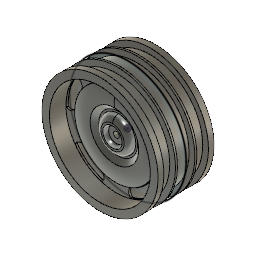
Primeira Modelagem (Autodesk Fusion 360 design; units mm, degrees)
Autodesk Fusion 360 part; units mm, degrees
sketch "Sketch1" plane through (0, 0, 0) normal (0, 1, 0) x (1, 0, 0)
  circle A0 centre (0, 0) radius 3
  dimension "d1" = 6
  constraint coincident A0.centre origin
  measures "d1" diameter of A0
sketch "Sketch1 (2)" plane through (0, 0, 0) normal (1, 0, 0) x (0, 1, 0) in component "roda"
  line L0 (0, -3) -> (0, 3)
  line L1 (-1.4737, 3.362) -> (1.4263, 3.362)
  line L2 (0, 2.7) -> (0.45, 2.7)
  line L3 (0.45, 2.7) -> (0.45, 3)
  line L4 (0.45, 3) -> (0.55, 3)
  line L5 (0.55, 3) -> (0.55, 2.7)
  line L6 (0.55, 2.7) -> (1.15, 2.7)
  line L7 (1.15, 2.7) -> (1.15, 3)
  line L8 (1.15, 3) -> (1.45, 3)
  line L9 (1.45, 3) -> (1.45, 2.6)
  line L10 (1.45, 2.6) -> (0, 2.6)
  line L11 (-0.45, 2.7) -> (-0.45, 3)
  line L12 (-0.45, 3) -> (-0.55, 3)
  line L13 (-0.55, 3) -> (-0.55, 2.7)
  line L14 (-0.55, 2.7) -> (-1.15, 2.7)
  line L15 (-1.15, 2.7) -> (-1.15, 3)
  line L16 (-1.15, 3) -> (-1.45, 3)
  line L17 (-1.45, 3) -> (-1.45, 2.6)
  line L18 (0, 2.7) -> (-0.45, 2.7)
  line L19 (-1.45, 2.6) -> (0, 2.6)
  dimension "d5" = 2.9
  dimension "d6" = 0.45
  dimension "d7" = 0.3
  dimension "d8" = 0.1
  dimension "d9" = 0.3
  dimension "d10" = 0.6
  dimension "d11" = 0.3
  dimension "d12" = 0.3
  dimension "d13" = 0.4
  dimension "d14" = 1.45
  constraint horizontal L1
  constraint coincident L0 L2.start
  constraint perpendicular L0 L2
  constraint perpendicular L2 L3
  constraint perpendicular L3 L4
  constraint perpendicular L4 L5
  constraint perpendicular L5 L6
  constraint perpendicular L6 L7
  constraint perpendicular L7 L8
  constraint perpendicular L8 L9
  constraint perpendicular L0 L10
  constraint symmetric L0 L2.start L18.start
  constraint symmetric L0 L2.end L11.start
  constraint symmetric L0 L3.end L11.end
  constraint symmetric L0 L4.end L12.end
  constraint symmetric L0 L5.end L13.end
  constraint symmetric L0 L6.end L14.end
  constraint symmetric L0 L7.end L15.end
  constraint symmetric L0 L8.end L16.end
  constraint symmetric L0 L9.end L17.end
  constraint symmetric L0 L10.end L19.end
  measures "d5" distance of L1.start L1.end
  measures "d6" distance of L2.start L2.end
  measures "d7" distance of L2.end L3.end
  measures "d8" distance of L3.end L4.end
  measures "d9" distance of L4.end L5.end
  measures "d10" distance of L5.end L6.end
  measures "d11" distance of L6.end L7.end
  measures "d12" distance of L7.end L8.end
  measures "d13" distance of L8.end L9.end
  measures "d14" distance of L9.end L10.end
revolve "Revolve1" add sketch "Sketch1 (2)" angle 360 about axis through (0, 1.75, 0) along (0, 1, 0) contours L0 L11 L12 L13 L14 L15 L16 L17 L18 L19 | L0 L2 L3 L4 L5 L6 L7 L8 L9 L10 picked at (-1.35, 2.7667) picked at (1.35, 2.7667) in component "roda"
sketch "Sketch2" plane through (0, 0, 0) normal (1, 0, 0) x (0, 1, 0) in component "roda"
  line L0 (-1.4529, 3.0989) -> (-0.6529, 3.0989)
  line L1 (-0.6, 2.6) -> (-0.6, 2.1)
  line L2 (-0.65, 2.1) -> (-0.65, 1.3) construction
  line L3 (-0.65, 2.1) -> (-0.6, 2.1)
  spline S0 degree 5 poles (-0.7, 1.25) (-0.7009, 1.2686) (-0.7026, 1.3058) (-0.7045, 1.3611) (-0.7061, 1.4339) (-0.7064, 1.5234) (-0.7046, 1.6112) (-0.7007, 1.6972) (-0.6947, 1.7813) (-0.6864, 1.8635) (-0.6762, 1.944) (-0.6666, 2.0071) (-0.6586, 2.0538) (-0.6529, 2.0847) (-0.65, 2.1) knots 0 0 0 0 0 0 0.1 0.2 0.3 0.4 0.5 0.6 0.7 0.8 0.9 1 1 1 1 1 1
  line L4 (-1.6, 3) -> (-1.6, 0) construction
  line L5 (-0.7, 1.25) -> (-0.5001, 1.0001)
  line L6 (-0.5001, 1.0001) -> (-0.5001, 0.9001)
  spline S1 degree 5 poles (-0.5001, 0.9001) (-0.5099, 0.8979) (-0.5291, 0.8931) (-0.557, 0.885) (-0.5921, 0.8722) (-0.6325, 0.8525) (-0.6689, 0.8289) (-0.7011, 0.8011) (-0.7289, 0.7689) (-0.7524, 0.7324) (-0.7721, 0.6921) (-0.7849, 0.6569) (-0.793, 0.629) (-0.7978, 0.6098) (-0.8, 0.6) knots 0 0 0 0 0 0 0.1 0.2 0.3 0.4 0.5 0.6 0.7 0.8 0.9 1 1 1 1 1 1
  line L7 (-0.8, 0.6) -> (-0.8, 0.5)
  spline S2 degree 5 poles (-0.8, 0.5) (-0.7942, 0.4984) (-0.7829, 0.4952) (-0.7663, 0.4902) (-0.7451, 0.4834) (-0.7203, 0.4745) (-0.6973, 0.4652) (-0.6763, 0.4554) (-0.6573, 0.4452) (-0.6403, 0.4345) (-0.6251, 0.4234) (-0.6143, 0.4142) (-0.6069, 0.4072) (-0.6022, 0.4024) (-0.6, 0.4) knots 0 0 0 0 0 0 0.1 0.2 0.3 0.4 0.5 0.6 0.7 0.8 0.9 1 1 1 1 1 1
  line L8 (-0.5974, -0.1475) -> (-0.5974, 0.1525) construction
  line L9 (-0.6, 0.4) -> (-0.6, 0.153)
  line L10 (-0.6, 2.6) -> (-0.6, 2.6261)
  line L11 (-0.6, 2.6261) -> (-0.5, 2.6261)
  line L12 (-0.5, 2.6261) -> (-0.5, 2)
  line L13 (-0.5, 2) -> (-0.55, 2)
  line L14 (-0.6, 0.153) -> (-0.25, 0.153)
  line L15 (-0.25, 0.153) -> (-0.25, 0.25)
  line L16 (-0.25, 0.25) -> (-0.4, 0.25)
  spline S3 degree 5 poles (-0.4, 0.25) (-0.3945, 0.2578) (-0.3852, 0.2732) (-0.3761, 0.2951) (-0.3736, 0.3222) (-0.3865, 0.3525) (-0.4146, 0.3797) (-0.4554, 0.4045) (-0.5048, 0.428) (-0.5565, 0.4524) (-0.6032, 0.4797) (-0.6379, 0.5119) (-0.6552, 0.55) (-0.6527, 0.5944) (-0.6318, 0.6435) (-0.5968, 0.6948) (-0.5536, 0.7453) (-0.5086, 0.792) (-0.4675, 0.8321) (-0.4343, 0.864) (-0.411, 0.8866) (-0.401, 0.8971) (-0.3986, 0.9006) (-0.3992, 0.901) (-0.4, 0.9007) knots 0 0 0 0 0 0 0.05 0.1 0.15 0.2 0.25 0.3 0.35 0.4 0.45 0.5 0.55 0.6 0.65 0.7 0.75 0.8 0.85 0.9 0.95 1 1 1 1 1 1
  spline S4 degree 5 poles (-0.4, 0.9007) (-0.3959, 0.9116) (-0.3884, 0.9333) (-0.3789, 0.9653) (-0.3701, 1.007) (-0.3658, 1.0572) (-0.3688, 1.1054) (-0.3797, 1.1514) (-0.3988, 1.1952) (-0.4258, 1.2369) (-0.4602, 1.2765) (-0.493, 1.3068) (-0.5204, 1.3287) (-0.5399, 1.3429) (-0.55, 1.35) knots 0 0 0 0 0 0 0.1 0.2 0.3 0.4 0.5 0.6 0.7 0.8 0.9 1 1 1 1 1 1
  line L17 (-0.55, 2) -> (-0.55, 1.35)
  point P0 (-0.7, 1.7)
  point P1 (-0.7, 0.8)
  point P2 (-0.676, 0.4549)
  point P3 (-0.45, 0.4)
  point P4 (-0.65, 0.55)
  point P5 (-0.5, 0.8)
  point P6 (-0.3816, 1.1504)
  dimension "d16" = 0.8
  dimension "d17" = 0.5
  dimension "d18" = 0.8
  dimension "d19" = 0.05
  dimension "d20" = 3
  dimension "d21" = 0.32
  dimension "d22" = 0.1
  dimension "d23" = 0.1
  dimension "d24" = 0.3
  dimension "d25" = 0.247
  dimension "d26" = 0.6261
  dimension "d27" = 0.65
  constraint horizontal L0
  constraint vertical L1
  constraint vertical L2
  constraint perpendicular L1 L3
  constraint vertical L4
  constraint vertical L6
  constraint vertical L7
  constraint vertical L8
  constraint parallel L8 L9
  constraint parallel L1 L10
  constraint perpendicular L10 L11
  constraint perpendicular L11 L12
  constraint perpendicular L12 L13
  constraint perpendicular L8 L14
  constraint perpendicular L14 L15
  constraint perpendicular L15 L16
  constraint perpendicular L13 L17
  measures "d16" distance of L0.start L0.end
  measures "d17" distance of L1.start L1.end
  measures "d18" distance of L2.start L2.end
  measures "d19" distance of L2.start L1.end
  measures "d20" distance of L4.start L4.end
  measures "d21" distance of S0.start L5.end
  measures "d22" distance of L5.end L6.end
  measures "d23" distance of S1.end L7.end
  measures "d24" distance of L8.start L8.end
  measures "d25" distance of S2.end L9.end
  measures "d26" distance of L11.end L12.end
  measures "d27" distance of L13.end S4.end
revolve "Revolve2" add sketch "Sketch2" angle 360 about axis through (0, 1.75, 0) along (0, 1, 0) contours L1 L3 S0 L5 L6 S1 L7 S2 L9 L10 L11 L12 L13 L14 L15 L16 S3 S4 L17 picked at (-0.5506, 1.1718) in component "roda"
sketch "Sketch3" plane through (0, 0, 0) normal (0, 1, 0) x (1, 0, 0) in component "roda"
  line L0 (0, 0) -> (0, -3.2) construction
  spline S0 degree 5 poles (0, -2.1172) (0.0042, -2.1177) (0.0131, -2.1185) (0.0278, -2.1195) (0.0489, -2.1204) (0.0728, -2.1208) (0.0907, -2.1208) (0.1016, -2.1209) (0.1145, -2.1219) (0.1328, -2.1217) (0.1566, -2.1201) (0.1839, -2.1172) (0.212, -2.1136) (0.2389, -2.1098) (0.2639, -2.1058) (0.2877, -2.1019) (0.3109, -2.098) (0.3345, -2.0939) (0.3592, -2.0895) (0.3848, -2.0845) (0.4108, -2.0789) (0.4367, -2.0725) (0.4618, -2.0655) (0.4859, -2.0582) (0.5093, -2.0513) (0.5324, -2.0455) (0.5557, -2.0415) (0.5797, -2.0402) (0.6045, -2.042) (0.63, -2.0473) (0.6557, -2.0562) (0.681, -2.0685) (0.7053, -2.0839) (0.7282, -2.1017) (0.7494, -2.1213) (0.7687, -2.1419) (0.7862, -2.1626) (0.8018, -2.1831) (0.8156, -2.2029) (0.8274, -2.2225) (0.8374, -2.2421) (0.8454, -2.2626) (0.8514, -2.2846) (0.8553, -2.3086) (0.8572, -2.335) (0.857, -2.364) (0.8552, -2.3895) (0.853, -2.4098) (0.8511, -2.4239) (0.85, -2.4311) knots 0 0 0 0 0 0 0.022222 0.044444 0.066667 0.088889 0.111111 0.133333 0.155556 0.177778 0.2 0.222222 0.244444 0.266667 0.288889 0.311111 0.333333 0.355556 0.377778 0.4 0.422222 0.444444 0.466667 0.488889 0.511111 0.533333 0.555556 0.577778 0.6 0.622222 0.644444 0.666667 0.688889 0.711111 0.733333 0.755556 0.777778 0.8 0.822222 0.844444 0.866667 0.888889 0.911111 0.933333 0.955556 0.977778 1 1 1 1 1 1
  spline S1 degree 5 poles (0, -2.5912) (0.0036, -2.5926) (0.0111, -2.5951) (0.0226, -2.5975) (0.0388, -2.5984) (0.0603, -2.5966) (0.0832, -2.5934) (0.1072, -2.5901) (0.1321, -2.5875) (0.1574, -2.5858) (0.1826, -2.5847) (0.2077, -2.5839) (0.2328, -2.5828) (0.2588, -2.5809) (0.2872, -2.5779) (0.3194, -2.5737) (0.3568, -2.5683) (0.4, -2.5615) (0.4487, -2.5532) (0.5015, -2.5433) (0.5564, -2.5319) (0.6112, -2.5189) (0.6637, -2.5044) (0.7121, -2.489) (0.7555, -2.4733) (0.7933, -2.4578) (0.8189, -2.4463) (0.8354, -2.4384) (0.8453, -2.4335) (0.85, -2.4311) knots 0 0 0 0 0 0 0.04 0.08 0.12 0.16 0.2 0.24 0.28 0.32 0.36 0.4 0.44 0.48 0.52 0.56 0.6 0.64 0.68 0.72 0.76 0.8 0.84 0.88 0.92 0.96 1 1 1 1 1 1
  spline S2 degree 5 poles (0, -2.1172) (-0.0042, -2.1177) (-0.0127, -2.1185) (-0.0253, -2.1193) (-0.042, -2.1197) (-0.0626, -2.1199) (-0.083, -2.1203) (-0.1033, -2.1212) (-0.1237, -2.1218) (-0.1444, -2.1213) (-0.1655, -2.1197) (-0.1874, -2.1171) (-0.2101, -2.1137) (-0.2337, -2.11) (-0.2582, -2.1061) (-0.2835, -2.1021) (-0.3093, -2.0981) (-0.3353, -2.0938) (-0.3614, -2.0893) (-0.3873, -2.0844) (-0.4127, -2.0788) (-0.4374, -2.0725) (-0.4615, -2.0655) (-0.485, -2.0583) (-0.5083, -2.0514) (-0.5316, -2.0455) (-0.5554, -2.0415) (-0.5798, -2.0402) (-0.6049, -2.042) (-0.6305, -2.0473) (-0.656, -2.0562) (-0.6811, -2.0685) (-0.7052, -2.0839) (-0.728, -2.1017) (-0.7492, -2.1213) (-0.7686, -2.1419) (-0.7861, -2.1626) (-0.8018, -2.1831) (-0.8156, -2.2029) (-0.8275, -2.2225) (-0.8375, -2.2421) (-0.8454, -2.2626) (-0.8514, -2.2846) (-0.8553, -2.3086) (-0.8572, -2.335) (-0.857, -2.364) (-0.8552, -2.3895) (-0.853, -2.4098) (-0.8511, -2.4239) (-0.85, -2.4311) knots 0 0 0 0 0 0 0.022222 0.044444 0.066667 0.088889 0.111111 0.133333 0.155556 0.177778 0.2 0.222222 0.244444 0.266667 0.288889 0.311111 0.333333 0.355556 0.377778 0.4 0.422222 0.444444 0.466667 0.488889 0.511111 0.533333 0.555556 0.577778 0.6 0.622222 0.644444 0.666667 0.688889 0.711111 0.733333 0.755556 0.777778 0.8 0.822222 0.844444 0.866667 0.888889 0.911111 0.933333 0.955556 0.977778 1 1 1 1 1 1
  line L1 (-0.1122, -2.1052) -> (0.1122, -2.1293)
  line L2 (0.8699, -2.2957) -> (0.8301, -2.5665)
  line L3 (0.1122, -2.1052) -> (-0.1122, -2.1293)
  line L4 (-0.8699, -2.2957) -> (-0.8301, -2.5665)
  spline S3 degree 5 poles (0, -2.5912) (-0.0036, -2.5926) (-0.0111, -2.5951) (-0.0226, -2.5975) (-0.0388, -2.5984) (-0.0603, -2.5966) (-0.0832, -2.5934) (-0.1072, -2.5901) (-0.1321, -2.5875) (-0.1574, -2.5858) (-0.1826, -2.5847) (-0.2077, -2.5839) (-0.2328, -2.5828) (-0.2588, -2.5809) (-0.2872, -2.5779) (-0.3194, -2.5737) (-0.3568, -2.5683) (-0.4, -2.5615) (-0.4487, -2.5532) (-0.5015, -2.5433) (-0.5564, -2.5319) (-0.6112, -2.5189) (-0.6637, -2.5044) (-0.7121, -2.489) (-0.7555, -2.4733) (-0.7933, -2.4578) (-0.8189, -2.4463) (-0.8354, -2.4384) (-0.8453, -2.4335) (-0.85, -2.4311) knots 0 0 0 0 0 0 0.04 0.08 0.12 0.16 0.2 0.24 0.28 0.32 0.36 0.4 0.44 0.48 0.52 0.56 0.6 0.64 0.68 0.72 0.76 0.8 0.84 0.88 0.92 0.96 1 1 1 1 1 1
  line L5 (-0.0741, -2.562) -> (0.0741, -2.6204)
  line L6 (0.7987, -2.4574) -> (0.9013, -2.4048)
  line L7 (0.0741, -2.562) -> (-0.0741, -2.6204)
  line L8 (-0.7987, -2.4574) -> (-0.9013, -2.4048)
  line L9 (0.0063, -2.1172) -> (-0.2063, -2.1248)
  line L10 (-0.0063, -2.1172) -> (0.2063, -2.1248)
  arc A0 (-0.155, -2.5875) -> (0.3214, -2.6043) centre (0.0895, -2.4182) cw
  point P0 (0.1, -2.121)
  point P1 (0.2033, -2.1147)
  point P2 (0.3277, -2.095)
  point P3 (0.4555, -2.0672)
  point P4 (0.5734, -2.041)
  point P5 (0.7, -2.0811)
  point P6 (0.8, -2.1811)
  point P7 (0.85, -2.2811)
  point P8 (0.1, -2.5912)
  point P9 (0.2197, -2.5833)
  point P10 (0.3752, -2.5653)
  point P11 (0.6553, -2.5063)
  point P12 (-0.1, -2.121)
  point P13 (-0.2033, -2.1147)
  point P14 (-0.3277, -2.095)
  point P15 (-0.4555, -2.0672)
  point P16 (-0.5734, -2.041)
  point P17 (-0.7, -2.0811)
  point P18 (-0.8, -2.1811)
  point P19 (-0.85, -2.2811)
  point P20 (-0.1, -2.5912)
  point P21 (-0.2197, -2.5833)
  point P22 (-0.3752, -2.5653)
  point P23 (-0.6553, -2.5063)
  constraint coincident L0.start origin
  constraint vertical L0
  constraint coincident L0 S0.start
  constraint coincident L0 S1.start
  constraint midpoint S0.start L1
  constraint midpoint S0.end L2
  constraint midpoint S1.start L5
  constraint midpoint S0.end L6
  constraint symmetric L0 P0 P12
  constraint symmetric L0 P1 P13
  constraint symmetric L0 P2 P14
  constraint symmetric L0 P3 P15
  constraint symmetric L0 P4 P16
  constraint symmetric L0 P5 P17
  constraint symmetric L0 P6 P18
  constraint symmetric L0 P7 P19
  constraint symmetric L0 S0.end S2.end
  constraint symmetric L0 S1.start S3.start
  constraint symmetric L0 P8 P20
  constraint symmetric L0 P9 P21
  constraint symmetric L0 P10 P22
  constraint symmetric L0 P11 P23
  constraint symmetric L0 L1.start L3.start
  constraint symmetric L0 L1.end L3.end
  constraint symmetric L0 L2.start L4.start
  constraint symmetric L0 L2.end L4.end
  constraint symmetric L0 L5.start L7.start
  constraint symmetric L0 L5.end L7.end
  constraint symmetric L0 L6.start L8.start
  constraint symmetric L0 L6.end L8.end
  constraint midpoint P12 L9
  constraint symmetric L0 L9.start L10.start
  constraint symmetric L0 L9.end L10.end
  constraint midpoint P0 L10
  constraint midpoint P0 A0
extrude "Extrude1" cut sketch "Sketch3" against normal blind 20 contours S1 S3 A0 | S2 L1 S3 L9 A0 | S0 S1 A0 | S0 L1 L10 A0 picked at (0.1281, -2.4359) picked at (-0.413, -2.3245) picked at (0.5821, -2.3419) picked at (0.0547, -2.1215) in component "roda"
pattern_circular "C-Pattern1" count 5 over 360 about axis through (0, 1.75, 0) along (0, 1, 0) of "Extrude1" in component "roda"
component "roda" placed x (1, 0, 0) y (0, 1, 0) z (0, 0, 1) at (0, 0, 0)
